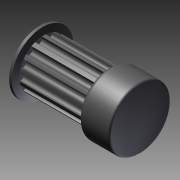
# Autodesk Inventor part: zrr_htd_3m15_0_17031400
Saved by Autodesk Inventor 2011 SP1 (Build 150282100, 282)
## iProperties
Created: 2018-07-07
Part Number: zrr_htd_3m15_0_17031400
Catalog Web Link: www.cadenas.de
Description: zrr_htd_3m15-HTD Pulleys Profile 3M, Timing Belt Width 15mm
Vendor: MAEDLER
Document SubType Name: Modeling
Designer: psAdmin
Manufacturer: MAEDLER
Mass: 9.4 g
Surface Area: 20.3953 cm^2
Volume: 3.43731 cm^3
Density: 1 g/cm^3
Category: PARTsolutions
Company: MAEDLER
Title: zrr_htd_3m15_0_17031400
Author: Cadenas PARTsolutions
Comments: HTD Pulleys Profile 3M, Timing Belt Width 15mm
PSOL_IDENT_0: {$CADENAS_DATA\23d-libs\maedler\antriebselemente\zahnriemenraeder_zahnriemen\zahnriemenraeder\htd-pr
PSOL_IDENT_1: ofil\zrr_htd_3m15.prj},197 {VTYP=3D},{NB=zrr_htd_3m15_0_17031400},{LINA=zrr_htd_3m15_0_17031400},{NN=
PSOL_IDENT_2: zrr_htd_3m15},{DATE=16.06.2017 10:47:49},{GEOMDATE=09.06.2016 09:07:07},{VERSION=},{LINEID=230},{LIN
PSOL_IDENT_3: ESUBID=-1},{WBVAR=BX}  {NB=zrr_htd_3m15_0_17031400},{LINA=zrr_htd_3m15_0_17031400},{KT=DUMMY},{ARTNR=
PSOL_IDENT_4: 17031400},{PDF=PDF Katalogseite},{AUSF=14-3M-15-0F},{MAT=Aluminium},{ZTL=3.000},{ZRB=15.000},{Z=14.0
PSOL_IDENT_5: 00},{AUS=0F},{ZS=12.610},{BS=16.000},{DO=13.370},{ND=16.000},{B=17.000},{L=26.000},{I=0.000},{VB=0.0
PSOL_IDENT_6: 00},{FB=6.000},{BX=0},{GEW=9.400},{ZT=1.200},{ZB=1.800},{T=0.000},{BB=1.000}
NN: zrr_htd_3m15
NT: HTD-Zahnriemenräder Profil 3M, Zahnriemenbreite 15mm
NB: zrr_htd_3m15_0_17031400
NBSYN: zrr_htd_3m15_$BX._$ARTNR.
LINA: zrr_htd_3m15_0_17031400
ARTNR: 17031400
PDF: PDF Katalogseite
AUSF: 14-3M-15-0F
MAT: Aluminium
ZTL: 3.000
ZRB: 15.000
Z: 14.000
AUS: 0F
ZS: 12.610
BS: 16.000
DO: 13.370
ND: 16.000
B: 17.000
L: 26.000
I: 0.000
VB: 0.000
FB: 6.000
BX: 0
GEW: 9.400
ZT: 1.200
ZB: 1.800
T: 0.000
BB: 1.000
SUPPLIER: MAEDLER
ARTICLENO: zrr_htd_3m15_0_17031400
BOMINFO: zrr_htd_3m15_0_17031400
CREATOR: CADENAS GmbH
Autodesk Inventor part; units mm, degrees
ref_plane "YZ Plane" through (0, 0, 0) normal (1, 0, 0) x (0, 1, 0)
ref_plane "XZ Plane" through (0, 0, 0) normal (0, 1, 0) x (-1, 0, 0)
ref_plane "XY Plane" through (0, 0, 0) normal (0, 0, 1) x (1, 0, 0)
sketch "Sketch_1" plane through (0, 0, 0) normal (0, 0, 1) x (1, 0, 0)
  line L0 (500, 0) -> (-500, 0)
  line L1 (0.2989, 0) -> (0.2989, 6.305)
  line L2 (0.2989, 6.305) -> (0, 8)
  line L3 (0, 8) -> (0.7011, 8)
  line L4 (0.7011, 8) -> (1, 6.305)
  line L5 (1, 6.305) -> (18, 6.305)
  line L6 (18, 6.305) -> (18, 7)
  arc A0 (19, 8) -> (18, 7) centre (19, 7) ccw
  line L7 (19, 8) -> (25.5, 8)
  arc A1 (26, 7.5) -> (25.5, 8) centre (25.5, 7.5) ccw
  line L8 (26, 7.5) -> (26, 0)
  line L9 (26, 0) -> (0.2989, 0)
  constraints: 20 end point, 4 point on circle, 2 centre point
revolve "Revolution1" add sketch "Sketch_1" angle 360 about axis through (500, 0, 0) along (1, 0, 0)
sketch "Sketch_2" plane through (1, 0, 0) normal (1, 0, 0) x (0, 0, -1)
  circle A0 centre (0, 0) radius 12.61
  arc A1 (-6.305, 0) -> (-6.2842, -0.5112) centre (0, 0) ccw
  line L0 (-6.2842, -0.5112) -> (-6.0547, -0.4588)
  arc A2 (-4.977, -1.136) -> (-6.0547, -0.4588) centre (-5.8544, -1.3362) ccw
  arc A3 (-5.6542, -2.2137) -> (-4.977, -1.136) centre (-5.8544, -1.3362) ccw
  line L1 (-5.6542, -2.2137) -> (-5.8837, -2.2661)
  arc A4 (-5.8837, -2.2661) -> (-5.6806, -2.7356) centre (0, 0) ccw
  arc A5 (-5.6806, -2.7356) -> (-5.4401, -3.1872) centre (0, 0) ccw
  line L2 (-5.4401, -3.1872) -> (-5.256, -3.0404)
  arc A6 (-3.9912, -3.1829) -> (-5.256, -3.0404) centre (-4.6949, -3.7441) ccw
  arc A7 (-4.1338, -4.4477) -> (-3.9912, -3.1829) centre (-4.6949, -3.7441) ccw
  line L3 (-4.1338, -4.4477) -> (-4.3178, -4.5945)
  arc A8 (-4.3178, -4.5945) -> (-3.9311, -4.9294) centre (0, 0) ccw
  arc A9 (-3.9311, -4.9294) -> (-3.5185, -5.2319) centre (0, 0) ccw
  line L4 (-3.5185, -5.2319) -> (-3.4163, -5.0198)
  arc A10 (-2.215, -4.5994) -> (-3.4163, -5.0198) centre (-2.6055, -5.4103) ccw
  arc A11 (-1.7946, -5.8008) -> (-2.215, -4.5994) centre (-2.6055, -5.4103) ccw
  line L5 (-1.7946, -5.8008) -> (-1.8968, -6.0129)
  arc A12 (-1.8968, -6.0129) -> (-1.403, -6.1469) centre (0, 0) ccw
  arc A13 (-1.403, -6.1469) -> (-0.9, -6.2404) centre (0, 0) ccw
  line L6 (-0.9, -6.2404) -> (-0.9, -6.005)
  arc A14 (0, -5.105) -> (-0.9, -6.005) centre (0, -6.005) ccw
  arc A15 (0.9, -6.005) -> (0, -5.105) centre (0, -6.005) ccw
  line L7 (0.9, -6.005) -> (0.9, -6.2404)
  arc A16 (0.9, -6.2404) -> (1.403, -6.1469) centre (0, 0) ccw
  arc A17 (1.403, -6.1469) -> (1.8968, -6.0129) centre (0, 0) ccw
  line L8 (1.8968, -6.0129) -> (1.7946, -5.8008)
  arc A18 (2.215, -4.5994) -> (1.7946, -5.8008) centre (2.6055, -5.4103) ccw
  arc A19 (3.4163, -5.0198) -> (2.215, -4.5994) centre (2.6055, -5.4103) ccw
  line L9 (3.4163, -5.0198) -> (3.5185, -5.2319)
  arc A20 (3.5185, -5.2319) -> (3.9311, -4.9294) centre (0, 0) ccw
  arc A21 (3.9311, -4.9294) -> (4.3178, -4.5945) centre (0, 0) ccw
  line L10 (4.3178, -4.5945) -> (4.1338, -4.4477)
  arc A22 (3.9912, -3.1829) -> (4.1338, -4.4477) centre (4.6949, -3.7441) ccw
  arc A23 (5.256, -3.0404) -> (3.9912, -3.1829) centre (4.6949, -3.7441) ccw
  line L11 (5.256, -3.0404) -> (5.4401, -3.1872)
  arc A24 (5.4401, -3.1872) -> (5.6806, -2.7356) centre (0, 0) ccw
  arc A25 (5.6806, -2.7356) -> (5.8837, -2.2661) centre (0, 0) ccw
  line L12 (5.8837, -2.2661) -> (5.6542, -2.2137)
  arc A26 (4.977, -1.136) -> (5.6542, -2.2137) centre (5.8544, -1.3362) ccw
  arc A27 (6.0547, -0.4588) -> (4.977, -1.136) centre (5.8544, -1.3362) ccw
  line L13 (6.0547, -0.4588) -> (6.2842, -0.5112)
  arc A28 (6.2842, -0.5112) -> (6.305, 0) centre (0, 0) ccw
  arc A29 (6.305, 0) -> (6.2842, 0.5112) centre (0, 0) ccw
  line L14 (6.2842, 0.5112) -> (6.0547, 0.4588)
  arc A30 (4.977, 1.136) -> (6.0547, 0.4588) centre (5.8544, 1.3362) ccw
  arc A31 (5.6542, 2.2137) -> (4.977, 1.136) centre (5.8544, 1.3362) ccw
  line L15 (5.6542, 2.2137) -> (5.8837, 2.2661)
  arc A32 (5.8837, 2.2661) -> (5.6806, 2.7356) centre (0, 0) ccw
  arc A33 (5.6806, 2.7356) -> (5.4401, 3.1872) centre (0, 0) ccw
  line L16 (5.4401, 3.1872) -> (5.256, 3.0404)
  arc A34 (3.9912, 3.1829) -> (5.256, 3.0404) centre (4.6949, 3.7441) ccw
  arc A35 (4.1338, 4.4477) -> (3.9912, 3.1829) centre (4.6949, 3.7441) ccw
  line L17 (4.1338, 4.4477) -> (4.3178, 4.5945)
  arc A36 (4.3178, 4.5945) -> (3.9311, 4.9294) centre (0, 0) ccw
  arc A37 (3.9311, 4.9294) -> (3.5185, 5.2319) centre (0, 0) ccw
  line L18 (3.5185, 5.2319) -> (3.4163, 5.0198)
  arc A38 (2.215, 4.5994) -> (3.4163, 5.0198) centre (2.6055, 5.4103) ccw
  arc A39 (1.7946, 5.8008) -> (2.215, 4.5994) centre (2.6055, 5.4103) ccw
  line L19 (1.7946, 5.8008) -> (1.8968, 6.0129)
  arc A40 (1.8968, 6.0129) -> (1.403, 6.1469) centre (0, 0) ccw
  arc A41 (1.403, 6.1469) -> (0.9, 6.2404) centre (0, 0) ccw
  line L20 (0.9, 6.2404) -> (0.9, 6.005)
  arc A42 (0, 5.105) -> (0.9, 6.005) centre (0, 6.005) ccw
  arc A43 (-0.9, 6.005) -> (0, 5.105) centre (0, 6.005) ccw
  line L21 (-0.9, 6.005) -> (-0.9, 6.2404)
  arc A44 (-0.9, 6.2404) -> (-1.403, 6.1469) centre (0, 0) ccw
  arc A45 (-1.403, 6.1469) -> (-1.8968, 6.0129) centre (0, 0) ccw
  line L22 (-1.8968, 6.0129) -> (-1.7946, 5.8008)
  arc A46 (-2.215, 4.5994) -> (-1.7946, 5.8008) centre (-2.6055, 5.4103) ccw
  arc A47 (-3.4163, 5.0198) -> (-2.215, 4.5994) centre (-2.6055, 5.4103) ccw
  line L23 (-3.4163, 5.0198) -> (-3.5185, 5.2319)
  arc A48 (-3.5185, 5.2319) -> (-3.9311, 4.9294) centre (0, 0) ccw
  arc A49 (-3.9311, 4.9294) -> (-4.3178, 4.5945) centre (0, 0) ccw
  line L24 (-4.3178, 4.5945) -> (-4.1338, 4.4477)
  arc A50 (-3.9912, 3.1829) -> (-4.1338, 4.4477) centre (-4.6949, 3.7441) ccw
  arc A51 (-5.256, 3.0404) -> (-3.9912, 3.1829) centre (-4.6949, 3.7441) ccw
  line L25 (-5.256, 3.0404) -> (-5.4401, 3.1872)
  arc A52 (-5.4401, 3.1872) -> (-5.6806, 2.7356) centre (0, 0) ccw
  arc A53 (-5.6806, 2.7356) -> (-5.8837, 2.2661) centre (0, 0) ccw
  line L26 (-5.8837, 2.2661) -> (-5.6542, 2.2137)
  arc A54 (-4.977, 1.136) -> (-5.6542, 2.2137) centre (-5.8544, 1.3362) ccw
  arc A55 (-6.0547, 0.4588) -> (-4.977, 1.136) centre (-5.8544, 1.3362) ccw
  line L27 (-6.0547, 0.4588) -> (-6.2842, 0.5112)
  arc A56 (-6.2842, 0.5112) -> (-6.305, 0) centre (0, 0) ccw
  constraints: 112 point on circle, 57 centre point, 56 end point
extrude "Extrusion1" cut sketch "Sketch_2" along normal blind 17
body "Solid1"
